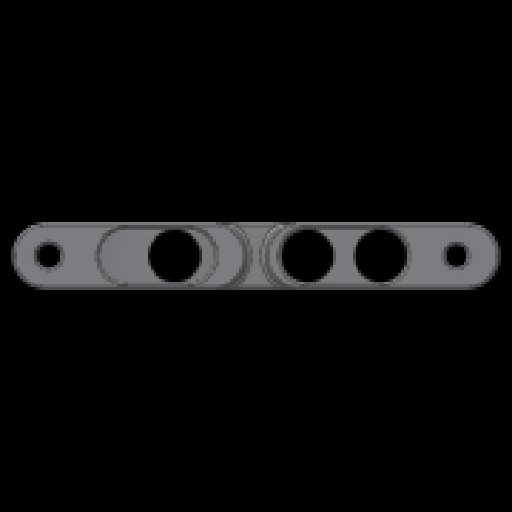
# Autodesk Inventor part: PrimeSenseCarmine1.09-Cover
Saved by Autodesk Inventor 2025.2 (Build 292293000, 293)
## iProperties
Created: 2024-11-08
Part Number: PrimeSenseCarmine1.09-Cover
Material: Generic
Document SubType Name: Modeling
Designer: valer
Density: 1 g/cm^3
Appearance: Default
Author: valer
Autodesk Inventor part; units mm, degrees
ref_plane "YZ Plane" through (0, 0, 0) normal (1, 0, 0) x (0, 1, 0)
ref_plane "XZ Plane" through (0, 0, 0) normal (0, 1, 0) x (-1, 0, 0)
ref_plane "XY Plane" through (0, 0, 0) normal (0, 0, 1) x (1, 0, 0)
sketch "Sensor" plane through (0, 0, 0) normal (0, 0, 1) x (1, 0, 0)
  circle A0 centre (19, 0) radius 8.875
  circle A1 centre (46, 0) radius 8.875
  circle A2 centre (-30, 0) radius 8.875
  circle A3 centre (-76.5, 0) radius 4.375
  line L0 (-90, 12.415) -> (90, 12.415)
  line L1 (90, 12.415) -> (90, -12.415)
  line L2 (90, -12.415) -> (-90, -12.415)
  line L3 (-90, -12.415) -> (-90, 12.415)
  line L4 (-90, 0) -> (90, 0) construction
  arc A4 (-77.585, 12.415) -> (-77.585, -12.415) centre (-77.585, 0) ccw
  arc A5 (77.585, -12.415) -> (77.585, 12.415) centre (77.585, 0) ccw
  circle A6 centre (74, 0) radius 4
  point P0 (0, 0)
  point P1 (0, 0)
  dimension "d0" = 17.75
  dimension "d1" = 180
  dimension "d2" = 24.83
  dimension "d3" = 8.75
  dimension "d4" = 46
  dimension "d5" = 27
  dimension "d6" = 30
  dimension "d7" = 13.5
  dimension "d8" = 16
  dimension "d9" = 8
  constraints: 8 end point, 7 centre point, 4 point on circle, 4 point on line, 4 tangent, 2 equal radius, 2 midpoint, 2 parallel, 1 coincident, 1 horizontal, 1 perpendicular, 11 other
  measures "d0" diameter of A0
  measures "d1" distance of L0.start L0.end
  measures "d2" distance of L2.end L0.start
  measures "d3" diameter of A3
  measures "d4" distance of point (0, 0) A1.centre
  measures "d5" distance of A1.centre A0.centre
  measures "d6" distance of point (0, 0) A2.centre
  measures "d7" distance from line of A3.centre L3
  measures "d8" distance from line of L1 A6.centre
  measures "d9" diameter of A6
extrude "SensorFeature" add sketch "Sensor" along normal blind 35.94 contours L0 A5 L2 A4
sketch "Sketch2" plane through (0, 0, 0) normal (0, 0, -1) x (-1, 0, 0)
  line L0 (-77.585, 12.415) -> (77.585, 12.415) projected
  arc A0 (-77.585, 12.415) -> (-77.585, -12.415) centre (-77.585, 0) ccw projected
  line L1 (77.585, -12.415) -> (-77.585, -12.415) projected
  arc A1 (77.585, -12.415) -> (77.585, 12.415) centre (77.585, 0) ccw projected
  point P0 (0, 0)
extrude "Extrusion2" add sketch "Sketch2" against normal blind 10
chamfer "Chamfer1" distance 4 angle 45 4 edges at (0, 12.415, 0) (-90, 0, 0) (0, -12.415, 0) (90, 0, 0)
sketch "Sketch7" plane through (0, 0, 35.94) normal (0, 0, 1) x (1, 0, 0)
  circle A0 centre (-30, 0) radius 8.875 construction
  circle A1 centre (19, 0) radius 8.875 construction
  circle A2 centre (46, 0) radius 8.875 construction
  circle A3 centre (-25, 0) radius 10
  line L0 (-25, 0) -> (-30, 0)
  circle A4 centre (-48, 0) radius 10
  line L1 (-48, 0) -> (-30, 0) construction
  line L2 (-48, 10) -> (-25, 10)
  line L3 (-48, -10) -> (-25, -10)
  circle A5 centre (19, 0) radius 10
  circle A6 centre (46, 0) radius 10
  line L4 (19, 10) -> (46, 10)
  line L5 (19, -10) -> (46, -10)
  point P0 (0, 0)
  dimension "d29" = 20
  dimension "d30" = 5
  dimension "d31" = 18
  constraints: 12 end point, 8 point on circle, 6 tangent, 4 centre point, 3 equal radius, 2 coincident, 1 collinear, 1 horizontal, 1 parallel
  measures "d29" diameter of A3
  measures "d30" distance of L0.start L0.end
  measures "d31" distance of L1.start L0.end
extrude "Extrusion6" cut sketch "Sketch7" against normal blind 3
chamfer "Chamfer2" distance 1 angle 45 5 edges at (-80.875, 0, 35.94) (70, 0, 35.94) (37.125, 0, 32.94) (10.125, 0, 32.94) (-38.875, 0, 32.94)
sketch "Sketch8" plane through (0, 0, 35.94) normal (0, 0, 1) x (1, 0, 0)
  circle A0 centre (16, 0) radius 12.415
  line L0 (0, 0) -> (90, 0) construction
  arc A1 (77.585, -12.415) -> (77.585, 12.415) centre (77.585, 0) ccw projected
  line L1 (77.585, 12.415) -> (-77.585, 12.415) construction
  line L2 (0, 0) -> (0, 12.415) construction
  line L3 (-77.585, 12.415) -> (77.585, 12.415) projected
  circle A2 centre (-16, 0) radius 12.415
  arc A3 (77.585, -12.415) -> (77.585, 12.415) centre (77.585, 0) ccw projected
  line L4 (16, 12.415) -> (77.585, 12.415)
  line L5 (16, -12.415) -> (77.585, -12.415)
  arc A4 (-77.585, 12.415) -> (-77.585, -12.415) centre (-77.585, 0) ccw projected
  line L6 (-77.585, 12.415) -> (-16, 12.415)
  line L7 (-77.585, -12.415) -> (-16, -12.415)
  line L8 (77.585, -12.415) -> (-77.585, -12.415) projected
  dimension "d45" = 16
  constraints: 12 end point, 5 point on circle, 5 tangent, 4 point on line, 3 horizontal, 2 centre point, 1 midpoint, 1 symmetric about line, 1 other
  measures "d45" distance of A0.centre L0.start
extrude "Extrusion7" cut sketch "Sketch8" against normal blind 2 contours A0 L8 A2 L3
fillet "Fillet4" radius 2 2 edges at (-3.585, 0, 33.94) (3.585, 0, 33.94)
fillet "Fillet5" radius 1 8 edges at (-15, 0, 35.94) (-36.5, -10, 35.94) (-58, 0, 35.94) (-36.5, 10, 35.94) (56, 0, 35.94) (32.5, -10, 35.94) (9, 0, 35.94) (32.5, 10, 35.94)
fillet "Fillet6" radius 1 4 edges at (-3.585, 0, 35.94) (-90, 0, 35.94) (-46.7925, -12.415, 35.94) (-46.7925, 12.415, 35.94)
fillet "Fillet7" radius 1 4 edges at (90, 0, 35.94) (46.7925, -12.415, 35.94) (46.7925, 12.415, 35.94) (3.585, 0, 35.94)
fillet "Fillet8" radius 1 14 edges at (-13.9642, -11.9923, 35.7565) (-11.0734, -12.415, 34.2429) (0, -12.415, 33.94) (11.0734, -12.415, 34.2429) (13.7805, -12.4017, 35.1027) (13.9642, -11.9923, 35.7565) (-13.7805, -12.4017, 35.1027) (11.0734, 12.415, 34.2429) (13.7105, 12.4073, 35.0643) (13.9642, 11.9923, 35.7565) (-10.9962, 12.415, 34.2254) (-13.7105, 12.4073, 35.0643) (-13.9642, 11.9923, 35.7565) (0, 12.415, 33.94)
split "Sculpt2" plane through (0, 0, 24.84) removes the side toward (0, 0, -1)
ref_plane "Work Plane3" through (0, 0, 24.84) normal (0, 0, 1) x (1, 0, 0)
sketch "Sketch10" plane through (77.585, -12.415, 24.84) normal (0, 0, -1) x (-1, 0, 0)
  arc A0 (0, 24.83) -> (0, 0) centre (0, 12.415) ccw projected
  line L0 (155.17, 0) -> (0, 0) projected
  line L1 (0, 24.83) -> (155.17, 24.83) projected
  arc A1 (155.17, 0) -> (155.17, 24.83) centre (155.17, 12.415) ccw projected
  arc A2 (0, 23.37) -> (0, 1.46) centre (0, 12.415) ccw
  line L2 (0, 23.37) -> (155.17, 23.37)
  arc A3 (155.17, 1.46) -> (155.17, 23.37) centre (155.17, 12.415) ccw
  line L3 (155.17, 1.46) -> (0, 1.46)
  point P0 (77.585, 12.415)
  dimension "d63" = 1.46
  constraints: 4 end point, 4 point on circle, 2 centre point, 3 other
  measures "d63" distance between parallel lines of L0 L3
extrude "Extrusion9" cut sketch "Sketch10" against normal blind 8 contours L2 A3 L3 A2
body "Solid1"
